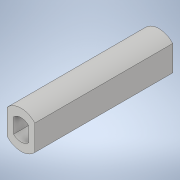
# Autodesk Inventor part: Motor Shaft Extension
Saved by Autodesk Inventor 2020.1 (Build 241239000, 239)
## iProperties
Created: 2019-11-05
Part Number: Motor Shaft Extension
Material: Generic
Document SubType Name: Modeling
Designer: ajtan
Density: 1 g/cm^3
Appearance: Default
Author: ajtan
Autodesk Inventor part; units mm, degrees
ref_plane "YZ Plane" through (0, 0, 0) normal (1, 0, 0) x (0, 1, 0)
ref_plane "XZ Plane" through (0, 0, 0) normal (0, 1, 0) x (-1, 0, 0)
ref_plane "XY Plane" through (0, 0, 0) normal (0, 0, 1) x (1, 0, 0)
sketch "Sketch1" plane through (0, 0, 0) normal (0, 0, 1) x (1, 0, 0)
  line L0 (2.4765, 2.4985) -> (2.4765, -2.4985)
  line L1 (-2.4765, 2.4985) -> (-2.4765, -2.4985)
  arc A0 (-2.4765, -2.4985) -> (2.4765, -2.4985) centre (0, 0) ccw
  arc A1 (2.4765, 2.4985) -> (-2.4765, 2.4985) centre (0, 0) ccw
  line L2 (4.572, 4.2217) -> (4.572, -4.2217)
  line L3 (-4.572, 4.2217) -> (-4.572, -4.2217)
  arc A2 (-4.572, -4.2217) -> (4.572, -4.2217) centre (0, 0) ccw
  arc A3 (4.572, 4.2217) -> (-4.572, 4.2217) centre (0, 0) ccw
  dimension "d2" = 2.4765
  dimension "d3" = 4.953
  dimension "d6" = 4.572
  dimension "d7" = 9.144
  dimension "d8" = 3.5179
  dimension "d9" = 3.5179
  dimension "d10" = 6.223
  dimension "d11" = 6.223
  constraints: 8 end point, 8 point on circle, 4 centre point, 4 vertical, 2 coincident, 1 parallel
  measures "d2" distance from line of point (0, 0) L0
  measures "d3" distance between parallel lines of L1 L0
  measures "d6" distance from line of point (0, 0) L2
  measures "d7" distance between parallel lines of L3 L2
  measures "d8" radius of A1
  measures "d9" radius of A0
  measures "d10" radius of A2
  measures "d11" radius of A3
extrude "Extrusion1" add sketch "Sketch1" along normal blind 45.72
equation "\"d2\" = 0.5 * d3"
equation "\"d6\" = 0.5 * d7"
body "Solid1"
